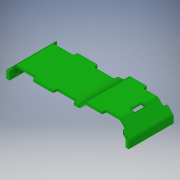
# Autodesk Inventor part: BODY_COVER
Saved by Autodesk Inventor 2017 (Build 210142000, 142)
## iProperties
Created: 2018-07-30
Part Number: BODY_COVER
Material: Generic
Document SubType Name: Modeling
Designer: Alexander Miller
Density: 1 g/cm^3
Appearance: Dark Green
Author: Alexander Miller
Autodesk Inventor part; units mm, degrees
ref_plane "YZ Plane" through (0, 0, 0) normal (1, 0, 0) x (0, 1, 0)
ref_plane "XZ Plane" through (0, 0, 0) normal (0, 1, 0) x (-1, 0, 0)
ref_plane "XY Plane" through (0, 0, 0) normal (0, 0, 1) x (1, 0, 0)
sketch "Sketch1" plane through (0, 0, 0) normal (0, 0, 1) x (1, 0, 0)
  line L0 (-79.35, 0) -> (-75.35, 0)
  line L1 (-75.35, 0) -> (-75.35, 13.07) construction
  line L2 (-75.35, 13.07) -> (24.587, 13.07) construction
  line L3 (24.587, 13.07) -> (24.587, 21.07) construction
  line L4 (24.587, 21.07) -> (56.587, 21.07) construction
  line L5 (56.587, 21.07) -> (56.587, 7.647) construction
  line L6 (56.587, 7.647) -> (75.35, 7.647) construction
  line L7 (75.35, 7.647) -> (75.35, 0) construction
  line L8 (75.35, 0) -> (79.35, 0)
  line L9 (79.35, 0) -> (79.35, 9.2396)
  line L10 (79.35, 9.2396) -> (64.0196, 24.57)
  line L11 (64.0196, 24.57) -> (22.5515, 24.57)
  line L12 (22.5515, 24.57) -> (14.5515, 16.57)
  line L13 (14.5515, 16.57) -> (-72.5352, 16.57)
  line L14 (-72.5352, 16.57) -> (-79.35, 9.7552)
  line L15 (-79.35, 9.7552) -> (-79.35, 0)
  line L16 (-75.35, 0) -> (75.35, 0) construction
  line L17 (-75.35, 0) -> (-75.35, 10.2197)
  line L18 (-75.35, 10.2197) -> (-71.4997, 14.07)
  line L19 (-71.4997, 14.07) -> (15.587, 14.07)
  line L20 (15.587, 14.07) -> (23.587, 22.07)
  line L21 (23.587, 22.07) -> (62.9841, 22.07)
  line L22 (62.9841, 22.07) -> (75.35, 9.7041)
  line L23 (75.35, 9.7041) -> (75.35, 0)
  arc A0 (64.35, 7.647) -> (56.587, 14.3585) centre (57.5673, 7.647) ccw construction
  point P0 (0, 0)
  point P1 (-77.35, 0)
  point P2 (0, 0)
  dimension "d0" = 158.7
  dimension "d1" = 4
  dimension "d2" = 4
  dimension "d3" = 103.937
  dimension "d4" = 22.763
  dimension "d5" = 7.647
  dimension "d6" = 13.07
  dimension "d7" = 21.07
  dimension "d9" = 2.5
  dimension "d10" = 2.5
  dimension "d11" = 2.5
  dimension "d12" = 2.5
  dimension "d13" = 15
  dimension "d14" = 1
  dimension "d15" = 1
  dimension "d16" = 1
  dimension "d19" = 45
  dimension "d20" = 135
  dimension "d21" = 135
  dimension "d22" = 2.5
  constraints: 48 end point, 9 perpendicular, 8 parallel, 5 point on line, 3 midpoint, 2 point on circle, 1 centre point, 1 coincident, 1 collinear, 1 horizontal, 1 horizontal alignment
  measures "d0" distance between parallel lines of L9 L15
  measures "d1" distance between parallel lines of L15 L1
  measures "d2" distance between parallel lines of L9 L7
  measures "d3" distance between parallel lines of L15 L3
  measures "d4" distance between parallel lines of L5 L9
  measures "d5" distance between parallel lines of L8 L6
  measures "d6" distance between parallel lines of L0 L2
  measures "d7" distance between parallel lines of L4 L8
  measures "d9" distance between parallel lines of L18 L14
  measures "d10" distance between parallel lines of L12 L20
  measures "d11" distance between parallel lines of L21 L11
  measures "d12" distance between parallel lines of L22 L10
  measures "d13" distance from line of L9 A0.start
  measures "d14" distance between parallel lines of L4 L21
  measures "d15" distance between parallel lines of L2 L19
  measures "d16" distance from line of L3 L20.end
  measures "d19" angle of L19 L20
  measures "d20" angle of L22 L23
  measures "d21" angle of L17 L18
  measures "d22" distance between parallel lines of L19 L13
extrude "Extrusion1" add sketch "Sketch1" along normal mid plane 58
sketch "Sketch2" plane through (-79.35, 0, 29) normal (0, -1, 0) x (1, 0, 0)
  line L0 (-31.74, -29) -> (190.44, -29) construction
  line L1 (153.35, -12) -> (121.85, -12) construction
  line L2 (121.85, -12) -> (121.85, 0) construction
  line L3 (121.85, 0) -> (153.35, 0) construction
  line L4 (153.35, 0) -> (153.35, -12) construction
  line L5 (89.6, -12) -> (58.1, -12) construction
  line L6 (58.1, -12) -> (58.1, 0) construction
  line L7 (58.1, 0) -> (89.6, 0) construction
  line L8 (89.6, 0) -> (89.6, -12) construction
  line L9 (36.85, -12) -> (5.35, -12) construction
  line L10 (5.35, -12) -> (5.35, 0) construction
  line L11 (5.35, 0) -> (36.85, 0) construction
  line L12 (36.85, 0) -> (36.85, -12) construction
  line L13 (85.35, -12) -> (62.35, -12) construction
  line L14 (62.35, -12) -> (62.35, 0) construction
  line L15 (62.35, 0) -> (85.35, 0) construction
  line L16 (85.35, 0) -> (85.35, -12) construction
  circle A0 centre (79.35, -6) radius 6 construction
  line L17 (150.6, -5) -> (124.6, -5)
  line L18 (124.6, -5) -> (124.6, 0)
  line L19 (124.6, 0) -> (150.6, 0)
  line L20 (150.6, 0) -> (150.6, -5)
  line L21 (86.85, -5) -> (60.85, -5)
  line L22 (60.85, -5) -> (60.85, 0)
  line L23 (60.85, 0) -> (86.85, 0)
  line L24 (86.85, 0) -> (86.85, -5)
  line L25 (34.1, -5) -> (8.1, -5)
  line L26 (8.1, -5) -> (8.1, 0)
  line L27 (8.1, 0) -> (34.1, 0)
  line L28 (34.1, 0) -> (34.1, -5)
  line L29 (0, 0) -> (0, -58) construction
  line L30 (158.7, -58) -> (158.7, 0) construction
  line L31 (0, -58) -> (158.7, -58) construction
  line L32 (158.7, -58) -> (158.7, 0) construction
  line L33 (158.7, 0) -> (0, 0) construction
  line L34 (0, 0) -> (0, -58) construction
  line L35 (58.1, -58) -> (89.6, -58) construction
  line L36 (62.35, -58) -> (85.35, -58) construction
  line L37 (150.6, -53) -> (124.6, -53)
  line L38 (124.6, -53) -> (124.6, -58)
  line L39 (124.6, -58) -> (150.6, -58)
  line L40 (150.6, -58) -> (150.6, -53)
  line L41 (86.85, -53) -> (60.85, -53)
  line L42 (60.85, -53) -> (60.85, -58)
  line L43 (60.85, -58) -> (86.85, -58)
  line L44 (86.85, -58) -> (86.85, -53)
  line L45 (34.1, -53) -> (8.1, -53)
  line L46 (8.1, -53) -> (8.1, -58)
  line L47 (8.1, -58) -> (34.1, -58)
  line L48 (34.1, -58) -> (34.1, -53)
  point P0 (79.35, -29)
  point P1 (4.35, -29)
  point P2 (73.85, -12)
  point P3 (73.85, -12)
  point P4 (73.85, -5)
  point P5 (21.1, -5)
  point P6 (21.1, -12)
  point P7 (137.6, -5)
  point P8 (137.6, -12)
  point P9 (4, 0)
  point P10 (34.1, -2.5)
  point P11 (60.85, -2.5)
  point P12 (86.85, -2.5)
  point P13 (124.6, -2.5)
  point P14 (121.85, -58)
  point P15 (36.85, -58)
  point P16 (79.35, -52)
  point P17 (73.85, -53)
  point P18 (21.1, -53)
  point P19 (137.6, -53)
  point P20 (34.1, -55.5)
  point P21 (60.85, -55.5)
  point P22 (86.85, -55.5)
  point P23 (124.6, -55.5)
  dimension "d31" = 31.5
  dimension "d32" = 23
  dimension "d33" = 12
  dimension "d34" = 26
  dimension "d35" = 5.35
  dimension "d36" = 5.35
  dimension "d37" = 5
  constraints: 92 end point, 26 symmetric about line, 16 parallel, 11 midpoint, 8 equal length, 8 horizontal, 8 perpendicular, 6 collinear, 4 vertical alignment, 3 horizontal alignment, 3 tangent, 1 centre point, 1 coincident
  measures "d31" distance of L1.start L1.end
  measures "d32" distance of L13.start L13.end
  measures "d33" distance of L1.end L2.end
  measures "d34" distance of L17.start L17.end
  measures "d35" distance between parallel lines of L4 L30
  measures "d36" distance between parallel lines of L10 L34
  measures "d37" distance of L25.end L26.end
extrude "Extrusion2" cut sketch "Sketch2" against normal through all
sketch "Sketch3" plane through (75.35, 0, 29) normal (0, -1, 0) x (1, 0, 0)
  line L0 (-10.5094, -22.214) -> (-15.068, -22.214)
  line L1 (-15.068, -22.214) -> (-15.068, -35.786)
  line L2 (-15.068, -35.786) -> (-10.5094, -35.786)
  line L3 (-10.5094, -35.786) -> (-10.5094, -22.214)
  line L4 (4, -58) -> (4, 0) projected
  point P0 (-75.35, -29)
  point P1 (4, -29)
  point P2 (-10.5094, -29)
  dimension "d38" = 19.068
  constraints: 8 end point, 2 midpoint, 2 parallel, 1 horizontal, 1 horizontal alignment, 1 perpendicular
  measures "d38" distance between parallel lines of L1 L4
extrude "Extrusion3" cut sketch "Sketch3" against normal through all
sketch "Sketch4" plane through (-75.35, 0, 29) normal (1, 0, 0) x (0, 0, -1)
  line L0 (8.65, 5.85) -> (14, 5.85)
  line L1 (14, 5.85) -> (14, 0.5)
  line L2 (14, 0.5) -> (8.65, 0.5)
  line L3 (8.65, 0.5) -> (8.65, 5.85)
  line L4 (44, 5.85) -> (49.35, 5.85)
  line L5 (49.35, 5.85) -> (49.35, 0.5)
  line L6 (49.35, 0.5) -> (44, 0.5)
  line L7 (44, 0.5) -> (44, 5.85)
  line L8 (14, 3.175) -> (44, 3.175) construction
  line L9 (58, 9.7552) -> (0, 9.7552) construction
  line L10 (58, 0) -> (0, 0) construction
  point P0 (29, 0)
  point P1 (29, 3.175)
  point P2 (29, 0)
  dimension "d41" = 5.35
  dimension "d42" = 0.5
  dimension "d43" = 30
  constraints: 18 end point, 5 parallel, 4 midpoint, 3 equal length, 2 horizontal, 2 perpendicular, 1 horizontal alignment, 1 vertical alignment
  measures "d41" distance of L0.start L0.end
  measures "d42" distance between parallel lines of L10 L2
  measures "d43" distance of L8.start L8.end
extrude "Extrusion4" cut sketch "Sketch4" against normal blind 3.35
sketch "Sketch5" plane through (75.35, 0, 29) normal (-1, 0, 0) x (0, 0, 1)
  line L0 (-49.35, 5.85) -> (-44, 5.85)
  line L1 (-44, 5.85) -> (-44, 0.5)
  line L2 (-44, 0.5) -> (-49.35, 0.5)
  line L3 (-49.35, 0.5) -> (-49.35, 5.85)
  line L4 (-14, 5.85) -> (-8.65, 5.85)
  line L5 (-8.65, 5.85) -> (-8.65, 0.5)
  line L6 (-8.65, 0.5) -> (-14, 0.5)
  line L7 (-14, 0.5) -> (-14, 5.85)
  line L8 (-44, 3.175) -> (-14, 3.175) construction
  line L9 (-58, 0) -> (0, 0) construction
  point P0 (-29, 0)
  point P1 (-29, 3.175)
  point P2 (-29, 0)
  dimension "d46" = 5.35
  dimension "d47" = 0.5
  dimension "d48" = 30
  constraints: 18 end point, 4 midpoint, 4 parallel, 3 equal length, 3 perpendicular, 2 horizontal, 1 horizontal alignment, 1 vertical alignment
  measures "d46" distance of L0.start L0.end
  measures "d47" distance between parallel lines of L9 L2
  measures "d48" distance of L8.start L8.end
extrude "Extrusion5" cut sketch "Sketch5" against normal blind 3.35
chamfer "Chamfer1" distance 1 angle 45 38 edges at (-18.5, 15.32, 24) (7.5, 15.32, 24) (-18.5, 15.32, 29) (7.5, 15.32, 29) (45.25, 23.32, 29) (45.25, 23.32, 24) (71.25, 15.5719, 24) (71.25, 15.5719, 29) (71.25, 15.5719, -24) (71.25, 15.5719, -29) (45.25, 23.32, -24) (45.25, 23.32, -29) (7.5, 15.32, -24) (7.5, 15.32, -29) (-18.5, 15.32, -24) (-18.5, 15.32, -29) (-45.25, 15.32, -29) (-45.25, 15.32, -24) (-71.25, 15.32, -24) (-71.25, 15.32, -29) (-71.25, 15.32, 29) (-71.25, 15.32, 24) (-45.25, 15.32, 24) (-45.25, 15.32, 29) (22.5515, 24.57, 0) (14.5515, 16.57, 0) (64.0196, 24.57, 15.393) (64.0196, 24.57, -15.393) (79.35, 9.2396, 0) (-72.5352, 16.57, 0) (-79.35, 9.7552, 0) (15.587, 14.07, 0) (23.587, 22.07, 0) (62.9841, 22.07, 15.393) (62.9841, 22.07, -15.393) (75.35, 9.7041, 0) (-75.35, 10.2197, 0) (-71.4997, 14.07, 0)
chamfer "Chamfer2" distance 1 angle 45 8 edges at (64.8406, 23.749, 0) (60.282, 24.57, 0) (60.282, 22.07, 0) (64.8406, 20.2135, 0) (63.8732, 24.2164, 6.786) (61.6508, 24.57, 6.786) (61.6508, 24.57, -6.786) (63.8732, 24.2164, -6.786)
equation "\"d2\" = d1"
equation "\"d9\" = shell"
equation "\"d10\" = shell"
equation "\"d11\" = shell"
equation "\"d12\" = shell"
equation "\"shell\" = 2.5"
equation "\"offset\" = 3"
body "Solid1"
